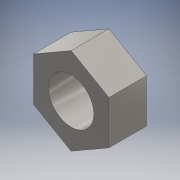
# Autodesk Inventor part: nut6mm
Saved by Autodesk Inventor 2016 (Build 200138000, 138)
## iProperties
Created: 2016-05-30
Part Number: nut6mm
Material: Stainless Steel
Document SubType Name: Modeling
Designer: Henrik Samuelsson
Density: 8 g/cm^3
Appearance: Semi-Polished
Author: Henrik Samuelsson
Autodesk Inventor part; units mm, degrees
ref_plane "YZ Plane" through (0, 0, 0) normal (1, 0, 0) x (0, 1, 0)
ref_plane "XZ Plane" through (0, 0, 0) normal (0, 1, 0) x (-1, 0, 0)
ref_plane "XY Plane" through (0, 0, 0) normal (0, 0, 1) x (1, 0, 0)
sketch "Sketch1" plane through (0, 0, 0) normal (0, 1, 0) x (-1, 0, 0)
  circle A0 centre (0, 0) radius 3
  line L0 (5, -2.8868) -> (0, -5.7735)
  line L1 (0, -5.7735) -> (-5, -2.8868)
  line L2 (-5, -2.8868) -> (-5, 2.8868)
  line L3 (-5, 2.8868) -> (0, 5.7735)
  line L4 (0, 5.7735) -> (5, 2.8868)
  line L5 (5, 2.8868) -> (5, -2.8868)
  dimension "d0" = 6
  dimension "d1" = 10
  constraints: 12 end point, 2 coincident, 1 centre point, 1 vertical, 13 other
  measures "d0" diameter of A0
  measures "d1" distance between parallel lines of L2 L5
extrude "Extrusion1" add sketch "Sketch1" along normal blind 5
body "Solid1"
